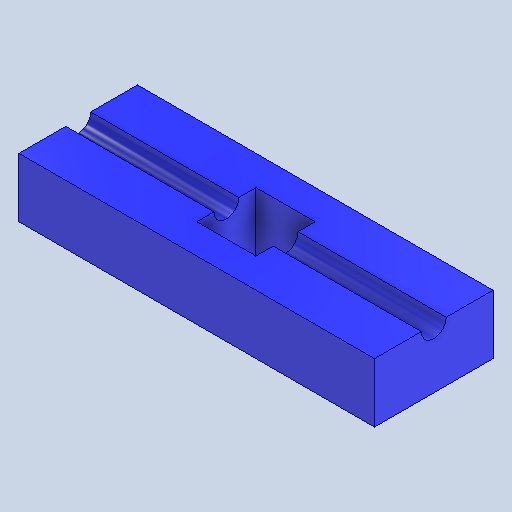
# Autodesk Inventor part: ball_loading_v1_3DP-circle_belt_zig
Saved by Autodesk Inventor 2025.1 (Build 291241000, 241)
## iProperties
Created: 2024-12-11
Part Number: ball_loading_v1_3DP-circle_belt_zig
Material: ABS プラスチック
Document SubType Name: Modeling
Designer: haruy
Density: 1.06 g/cm^3
Appearance: 青 - 壁塗料 - 光沢
Author: haruy
Autodesk Inventor part; units mm, degrees
ref_plane "YZ Plane" through (0, 0, 0) normal (1, 0, 0) x (0, 1, 0)
ref_plane "XZ Plane" through (0, 0, 0) normal (0, 1, 0) x (-1, 0, 0)
ref_plane "XY Plane" through (0, 0, 0) normal (0, 0, 1) x (1, 0, 0)
sketch "スケッチ1" plane through (0, 0, 0) normal (1, 0, 0) x (0, 1, 0)
  line L0 (0, 0) -> (10, 0)
  line L1 (10, 0) -> (10, -20)
  line L2 (10, -20) -> (0, -20)
  line L3 (0, -20) -> (0, 0)
  circle A0 centre (10, -10) radius 2.1
  point P0 (10, -12.1)
  point P1 (10, -7.9)
  dimension "d0" = 10
  dimension "d1" = 20
  dimension "d2" = 4.2
  dimension "d3" = 10
  dimension "d4" = 0
  constraints: 8 end point, 2 parallel, 1 centre point, 1 horizontal, 1 perpendicular
  measures "d0" distance of L1.end L2.end
  measures "d1" distance of L0.end L1.end
  measures "d2" diameter of A0
  measures "d3" distance from line of L0 A0.centre
  measures "d4" distance from line of L1 A0.centre
extrude "押し出し1" add sketch "スケッチ1" along normal blind 60 contours L0 L1 A0 L2 L3
sketch "スケッチ2" plane through (0, 10, -12.1) normal (0, 1, 0) x (1, 0, 0)
  line L0 (25, -7.1) -> (35, -7.1)
  line L1 (35, -7.1) -> (35, 2.9)
  line L2 (35, 2.9) -> (25, 2.9)
  line L3 (25, 2.9) -> (25, -7.1)
  line L4 (0, 7.9) -> (0, 0) projected
  line L5 (0, -12.1) -> (60, -12.1) projected
  dimension "d7" = 10
  dimension "d8" = 10
  dimension "d9" = 25
  dimension "d10" = 5
  constraints: 8 end point, 2 parallel, 1 horizontal, 1 perpendicular
  measures "d7" distance of L1.end L2.end
  measures "d8" distance of L0.end L1.end
  measures "d9" distance between parallel lines of L4 L3
  measures "d10" distance between parallel lines of L5 L0
extrude "押し出し2" cut sketch "スケッチ2" against normal through all
